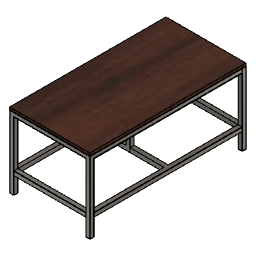
gyakorlati 12 asztal (Autodesk Fusion 360 design; units mm, degrees)
Autodesk Fusion 360 part; units mm, degrees
note: some values were not read from the file. Chosen so that the rebuilt part matches the saved one: which face or edge a step refers to. Set by a fixed rule: which sketch regions a step uses.
sketch "Sketch1" plane through (0, 0, 0) normal (0, 0, 1) x (1, 0, 0)
  line L0 (0, 0) -> (90, 0)
  line L1 (90, 0) -> (90, 180)
  line L2 (90, 180) -> (0, 180)
  line L3 (0, 180) -> (0, 0)
  line L4 (90, 180) -> (90, 185)
  line L5 (0, 180) -> (0, 185)
  line L6 (0, 185) -> (90, 185)
  line L7 (90, 180) -> (95, 180)
  line L8 (95, 180) -> (95, 0)
  line L9 (95, 0) -> (90, 0)
  line L10 (95, 5) -> (0, 5)
  line L11 (5, 0) -> (5, 185)
  line L12 (95, 180) -> (95, 185)
  line L13 (95, 185) -> (90, 185)
  line L14 (90, 95) -> (90, 97.5)
  line L15 (90, 95) -> (90, 92.5)
  line L16 (90, 92.5) -> (5, 92.5)
  line L17 (90, 97.5) -> (5, 97.5)
  line L18 (5, 97.5) -> (5, 92.5)
  line L19 (90, 92.5) -> (47.5, 92.5)
  line L20 (47.5, 92.5) -> (47.5, 97.5)
  line L21 (47.5, 97.5) -> (50, 97.5)
  line L22 (50, 97.5) -> (50, 92.5)
  line L23 (50, 92.5) -> (44.9965, 92.5)
  line L24 (44.9965, 97.5) -> (44.9965, 92.5)
  dimension "d7" = 5
  dimension "d12" = 2.5
  dimension "d13" = 2.5
  dimension "d16" = 42.5
  dimension "d17" = 2.5
  constraint coincident L0.start L3.end
  constraint horizontal L0
  constraint perpendicular L0 L1
  constraint perpendicular L1 L2
  constraint perpendicular L0 L3
  constraint perpendicular L2 L4
  constraint perpendicular L2 L5
  constraint perpendicular L4 L7
  constraint perpendicular L2 L8
  constraint perpendicular L1 L9
  constraint coincident L8 L10.start
  constraint coincident L3 L10.end
  constraint perpendicular L3 L10
  constraint coincident L0 L11.start
  constraint coincident L6 L11.end
  constraint perpendicular L6 L11
  constraint perpendicular L6 L12
  constraint perpendicular L4 L13
  constraint coincident L1 L14.start
  constraint midpoint L11 L16.end
  constraint coincident L11 L17.end
  constraint perpendicular L11 L17
  constraint parallel L11 L18
  constraint perpendicular L15 L19
  constraint midpoint L17 L20.end
  constraint perpendicular L20 L21
  constraint coincident L16 L22.end
  constraint perpendicular L16 L22
  constraint coincident L16 L23.end
  constraint coincident L17 L24.start
  constraint vertical L24
  measures "d7" distance of L7.end L12.end
  measures "d12" distance of L14.start L14.end
  measures "d13" distance of L14.start L15.end
  measures "d16" distance of L15.end L19.end
  measures "d17" distance of L20.end L21.end
extrude "Extrude1" add sketch "Sketch1" along normal blind 5 contours L0 L1 L10 L11 | L2 L3 L10 L11 L18 | L1 L7 L8 L10 L14 L15 | L2 L4 L6 L11 makes body 1 at (3.3333, 121.6667, 0)
extrude "Extrude2" add sketch "Sketch1" along normal blind 60 and the other way blind 20 separate body contours L1 L8 L9 L10 makes body 2
extrude "Extrude3" add sketch "Sketch1" along normal blind 60 and the other way blind 20 separate body contours L0 L3 L10 L11 | L2 L5 L6 L11 | L4 L7 L12 L13 makes body 3 at (93.3333, 185, 33.3333) makes body 4 at (1.6667, 185, 6.6667) makes body 5 at (3.3333, 5, 33.3333)
extrude "Extrude4" add sketch "Sketch1" along normal blind 5 separate body contours L11 L16 L17 L18 L24 | L1 L14 L15 L16 L17 L19 L22 | L16 L17 L20 L23 L24 | L16 L17 L19 L20 L21 L22 L23 makes body 6
extrude "Extrude5" cut 1 faces at (63.3333, 95, 5) along direction (0, 0, -1) blind 5 on bodies 6 bodies 6
extrude "Extrude6" add sketch "Sketch1" along normal blind 60 contours L16 L17 L20 L23 L24 | L16 L17 L19 L20 L21 L22 L23 bodies 6
extrude "Extrude7" add sketch "Sketch1" along normal blind 5 contours L11 L16 L17 L18 L24 | L1 L14 L15 L16 L17 L19 L22 bodies 6 2 3 4 5 1
sketch "Sketch2" plane through (0, 0, 60) normal (0, 0, 1) x (-1, 0, 0)
  line L0 (-5, 0) -> (-5, -5)
  line L1 (-5, -5) -> (0, -5)
  line L2 (0, -5) -> (0, 0)
  line L3 (0, 0) -> (-5, 0)
  line L4 (-5, 0) -> (-90, 0)
  line L5 (-90, 0) -> (-90, -5)
  line L6 (-90, -5) -> (-5, -5)
  line L7 (-5, 0) -> (-5, -5)
  line L8 (-95, -5) -> (-95, -180)
  line L9 (-90, -5) -> (-95, -5)
  line L10 (-90, -180) -> (-95, -180)
  line L11 (-90, -5) -> (-90, -180)
  line L12 (-5, -5) -> (-5, -180)
  line L13 (-5, -180) -> (-90, -180)
  line L14 (-5, -185) -> (-90, -185)
  line L15 (0, -180) -> (0, -5)
  line L16 (0, -180) -> (-5, -180)
  line L17 (-5, -180) -> (-5, -185)
  line L18 (-90, -180) -> (-90, -185)
  line L19 (-90, -92.5) -> (-90, -97.5)
  line L20 (-90, -97.5) -> (-5, -97.5)
  line L21 (-5, -92.5) -> (-90, -92.5)
  point P0 (-90, 0)
  point P1 (-90, -5)
  point P2 (-95, -5)
  point P3 (-95, -180)
  point P4 (-90, -180)
  point P5 (-90, -180)
  point P6 (-5, -180)
  point P7 (-5, -185)
  point P8 (-90, -185)
  point P9 (0, -180)
  dimension "d24" = 5
  constraint coincident L0.start L3.end
  constraint coincident P0 L4.end
  constraint coincident P1 L5.end
  constraint coincident L0.end L1.start
  constraint coincident P2 L8.start
  constraint coincident P3 L8.end
  constraint coincident P5 P4
  constraint coincident P6 L12.end
  constraint coincident P7 L14.start
  constraint coincident P8 L14.end
  constraint coincident P9 L15.start
  constraint coincident L1.end L2.start
  constraint midpoint L11 L19.start
  constraint coincident L11 L19.end
  constraint coincident L12 L20.end
  constraint perpendicular L12 L20
  constraint midpoint L12 L21.start
  measures "d24" distance of L19.start L19.end
extrude "Extrude8" add sketch "Sketch2" along normal blind 5 separate body contours L0 L4 L5 L6 L7 | L1 L12 L15 L16 | L8 L9 L10 L11 L19 | L11 L12 L19 L20 L21 | L13 L14 L17 L18 makes body 7 at (1.6667, 92.5, 60)
extrude "Extrude9" add 1 faces at (91.6667, 3.3333, 60) along direction (0, 0, 1) blind 5 on bodies 2 bodies 2 7
extrude "Extrude10" add 3 faces at (3.3333, 3.3333, 60) (93.3333, 183.3333, 60) (1.6667, 183.3333, 60) along direction (0, 0, 1) blind 5 on bodies 3 4 5 bodies 5 6 2 3 4
shell "Shell1" thickness 0.2 removed faces 4 at (3.3333, 3.3333, -20) at (93.3333, 183.3333, -20) at (91.6667, 3.3333, -20) at (1.6667, 183.3333, -20) on bodies 5
fillet "Fillet1" radius 0.3 17 edges at (5, 0, 20) (0, 0, 22.5) (4.8, 4.8, 20.1) (47.5, 0, 60) (90, 0, 20) (95, 0, 22.5) (94.8, 4.8, 20.1) (0.2, 4.8, 20.1) (90.2, 4.8, 20.1) (0, 180, 20) (5, 180, 20) (0.2, 184.8, 22.4) (4.8, 184.8, 20.1) (95, 185, 22.5) (90, 180, 20) (90.2, 184.8, 20.1) (95, 180, 20) on bodies 5
fillet "Fillet2" radius 0.3 1 edges at (4.8, 0.2, 20.1) on bodies 5
fillet "Fillet3" radius 0.3 4 edges at (90, 5, 20) (0, 5, 20) (0, 185, 22.5) (90, 185, 20) on bodies 5
fillet "Fillet4" radius 0.3 10 edges at (94.9121, 184.9121, 65) (92.35, 185, 65) (45.15, 185, 65) (0.0879, 184.9121, 65) (0, 92.5, 65) (0.0879, 0.0879, 65) (47.5, 0, 65) (94.9121, 0.0879, 65) (95, 90.15, 65) (95, 182.35, 65) on bodies 5
fillet "Fillet5" radius 0.3 6 edges at (47.35, 0.2, 60.2) (94.8, 92.25, 60.2) (94.8, 180.1, 60.2) (47.5, 185, 60) (90.15, 185, 60) (0.2, 92.35, 60.2) on bodies 5
fillet "Fillet6" radius 0.3 1 edges at (0, 92.5, 0) on bodies 6
fillet "Fillet7" radius 0.3 1 edges at (95, 92.5, 0) on bodies 6
fillet "Fillet8" radius 0.3 1 edges at (47.5, 0, 0) on bodies 6
fillet "Fillet9" radius 0.3 1 edges at (47.5, 0, 5) on bodies 6
fillet "Fillet10" radius 0.3 2 edges at (47.5, 185, 0) (47.5, 185, 5) on bodies 6
fillet "Fillet11" radius 0.3 4 edges at (44.9965, 97.5, 32.5) (50, 92.5, 32.5) (50, 97.5, 32.5) (44.9965, 92.5, 32.5) on bodies 6
ref_plane "WorkPlane1" through (0, 0, 65) normal (0, 0, 1) x (1, 0, 0) in component "teteje1"
sketch "Sketch1 (2)" plane through (0, 0, 65) normal (0, 0, 1) x (1, 0, 0) in component "teteje1"
  line L0 (0, 0) -> (94.7, 0.3)
  line L1 (94.7, 0.3) -> (94.7, 184.7)
  line L2 (94.7, 184.7) -> (0.3, 184.7)
  line L3 (0.3, 184.7) -> (0, 0)
  point P0 (94.7, 0.3)
  point P1 (94.7, 184.7)
  point P2 (0.3, 184.7)
  constraint coincident L0.start L3.end
  constraint coincident P0 L0.end
  constraint coincident P1 L1.end
  constraint coincident P2 L2.end
extrude "Extrude1'" add sketch "Sketch1 (2)" along normal blind 3 separate body makes body 8 in component "teteje1"
fillet "Fillet12" radius 0.3 1 edges at (95, 92.5, 5) on bodies 6
fillet "Fillet13" radius 0.3 1 edges at (0, 92.5, 5) on bodies 6
component "teteje1" placed x (1, 0, 0) y (0, 1, 0) z (0, 0, 1) at (0, 0, 0)
